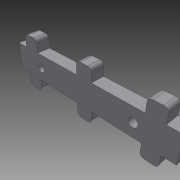
# Autodesk Inventor part: z_pulley_holder
Saved by Autodesk Inventor 2014 (Build 180170000, 170)
## iProperties
Created: 2014-04-04
Part Number: z_pulley_holder
Material: Plywood, Finish
Document SubType Name: Modeling
Designer: buben
Density: 0.552 g/cm^3
Appearance: Plywood - New
Author: buben
Autodesk Inventor part; units mm, degrees
ref_plane "YZ Plane" through (0, 0, 0) normal (1, 0, 0) x (0, 1, 0)
ref_plane "XZ Plane" through (0, 0, 0) normal (0, 1, 0) x (-1, 0, 0)
ref_plane "XY Plane" through (0, 0, 0) normal (0, 0, 1) x (1, 0, 0)
sketch "Sketch1" plane through (0, 0, 0) normal (0, 1, 0) x (-1, 0, 0)
  line L0 (0, 0) -> (-85, 0)
  line L1 (-85, 0) -> (-85, -13.5)
  line L2 (-85, -13.5) -> (0, -13.5)
  line L3 (0, -13.5) -> (0, 0)
  dimension "d0" = 85
  dimension "d1" = 13.5
  constraints: 8 end point, 2 parallel, 1 horizontal, 1 perpendicular
  measures "d0" distance of L0.start L0.end
  measures "d1" distance of L2.end L0.start
extrude "Extrusion1" add sketch "Sketch1" along normal blind 6.5
sketch "Sketch2" plane through (0, 6.5, 0) normal (0, 1, 0) x (1, 0, 0)
  line L0 (0, 0) -> (85, 0) projected
  line L1 (85, 0) -> (85, 13.5) projected
  line L2 (85, 13.5) -> (0, 13.5) projected
  line L3 (0, 13.5) -> (0, 0) projected
  line L4 (6, 13.5) -> (14, 13.5)
  line L5 (14, 13.5) -> (14, 18)
  line L6 (12, 20) -> (8, 20)
  line L7 (6, 18) -> (6, 13.5)
  line L8 (38.5, 13.5) -> (46.5, 13.5)
  line L9 (46.5, 13.5) -> (46.5, 18)
  line L10 (44.5, 20) -> (40.5, 20)
  line L11 (38.5, 18) -> (38.5, 13.5)
  line L12 (71, 13.5) -> (79, 13.5)
  line L13 (79, 13.5) -> (79, 18)
  line L14 (77, 20) -> (73, 20)
  line L15 (71, 18) -> (71, 13.5)
  line L16 (6, 0) -> (14, 0)
  line L17 (14, 0) -> (14, -4.5)
  line L18 (12, -6.5) -> (8, -6.5)
  line L19 (6, -4.5) -> (6, 0)
  line L20 (38.5, 0) -> (46.5, 0)
  line L21 (46.5, 0) -> (46.5, -4.5)
  line L22 (44.5, -6.5) -> (40.5, -6.5)
  line L23 (38.5, -4.5) -> (38.5, 0)
  line L24 (71, 0) -> (79, 0)
  line L25 (79, 0) -> (79, -4.5)
  line L26 (77, -6.5) -> (73, -6.5)
  line L27 (71, -4.5) -> (71, 0)
  arc A0 (8, 20) -> (6, 18) centre (8, 18) ccw
  arc A1 (14, 18) -> (12, 20) centre (12, 18) ccw
  arc A2 (40.5, 20) -> (38.5, 18) centre (40.5, 18) ccw
  arc A3 (46.5, 18) -> (44.5, 20) centre (44.5, 18) ccw
  arc A4 (73, 20) -> (71, 18) centre (73, 18) ccw
  arc A5 (79, 18) -> (77, 20) centre (77, 18) ccw
  arc A6 (6, -4.5) -> (8, -6.5) centre (8, -4.5) ccw
  arc A7 (12, -6.5) -> (14, -4.5) centre (12, -4.5) ccw
  arc A8 (38.5, -4.5) -> (40.5, -6.5) centre (40.5, -4.5) ccw
  arc A9 (44.5, -6.5) -> (46.5, -4.5) centre (44.5, -4.5) ccw
  arc A10 (71, -4.5) -> (73, -6.5) centre (73, -4.5) ccw
  arc A11 (77, -6.5) -> (79, -4.5) centre (77, -4.5) ccw
  line L28 (14, 15.75) -> (38.5, 15.75) construction
  line L29 (46.5, 15.75) -> (71, 15.75) construction
  dimension "d4" = 2
  dimension "d5" = 8
  dimension "d6" = 8
  dimension "d7" = 8
  dimension "d8" = 6.5
  dimension "d9" = 6.5
  dimension "d10" = 6
  dimension "d11" = 6
  constraints: 52 end point, 24 point on circle, 24 tangent, 12 centre point, 12 parallel, 11 collinear, 11 equal radius, 6 horizontal, 6 perpendicular, 6 point on line, 4 midpoint
  measures "d4" radius of A0
  measures "d5" distance between parallel lines of L5 L7
  measures "d6" distance between parallel lines of L9 L11
  measures "d7" distance between parallel lines of L13 L15
  measures "d8" distance between parallel lines of L4 L6
  measures "d9" distance between parallel lines of L0 L18
  measures "d10" distance between parallel lines of L3 L7
  measures "d11" distance between parallel lines of L1 L13
extrude "Extrusion2" add sketch "Sketch2" against normal blind 6.5 contours L0 L17 A7 L18 A6 L19 | L7 A0 L6 A1 L5 L2 | L0 L21 A9 L22 A8 L23 | L11 A2 L10 A3 L9 L2 | L0 L25 A11 L26 A10 L27 | L15 A4 L14 A5 L13 L2
sketch "Sketch4" plane through (0, 6.5, 0) normal (0, 1, 0) x (1, 0, 0)
  line L0 (85, 0) -> (85, 13.5) projected
  circle A0 centre (66.4711, 6.75) radius 2.25
  line L1 (46.5, 0) -> (71, 0) projected
  line L2 (85, 0) -> (0, -27.6346) construction
  line L3 (71, 13.5) -> (46.5, 13.5) projected
  line L4 (70.2271, -4.8028) -> (64.2766, 13.5) construction
  point P0 (85, 6.75)
  point P1 (0, 0)
  dimension "d14" = 4.5
  dimension "d18" = 18.01
  dimension "d19" = 15.534
  constraints: 4 end point, 3 point on line, 1 centre point, 1 horizontal alignment, 1 midpoint, 1 perpendicular, 1 vertical alignment
  measures "d14" diameter of A0
  measures "d18" angle of L1 L2
  measures "d19" distance of L0.start L4.start
extrude "Extrusion3" cut sketch "Sketch4" against normal through all
sketch "Sketch5" plane through (0, 6.5, 0) normal (0, 1, 0) x (1, 0, 0)
  circle A0 centre (66.4711, 6.75) radius 2.25 projected
  line L0 (85, 0) -> (85, 13.5) projected
  line L1 (0, 13.5) -> (0, 0) projected
  circle A1 centre (15.354, 6.75) radius 2.25
  point P0 (0, 6.75)
  dimension "d22" = 69.646
  constraints: 1 centre point, 1 equal radius, 1 horizontal alignment, 1 midpoint
  measures "d22" distance from line of A1.centre L0
extrude "Extrusion4" cut sketch "Sketch5" against normal through all contours A1
equation "\"d6\" = d5"
equation "\"d7\" = d6"
equation "\"d9\" = d8"
equation "\"d11\" = d10"
body "Solid1"
